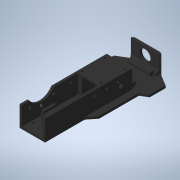
# Autodesk Inventor part: Griff_rechts
Saved by Autodesk Inventor 2021 (Build 250183000, 183)
## iProperties
Created: 2021-03-07
Part Number: Griff_rechts
Material: Generic
Document SubType Name: Modeling
Designer: Lukas
Density: 1 g/cm^3
Appearance: Default
Author: Lukas
Autodesk Inventor part; units mm, degrees
ref_plane "YZ Plane" through (0, 0, 0) normal (1, 0, 0) x (0, 1, 0)
ref_plane "XZ Plane" through (0, 0, 0) normal (0, 1, 0) x (-1, 0, 0)
ref_plane "XY Plane" through (0, 0, 0) normal (0, 0, 1) x (1, 0, 0)
sketch "Sketch27" plane through (0, 0, 0) normal (0, 1, 0) x (-1, 0, 0)
  line L0 (16, 72.5) -> (-16, 72.5)
  line L1 (-16, 72.5) -> (-16, -32.5)
  line L2 (16, -32.5) -> (16, 72.5)
  line L3 (16, -32.5) -> (32.5, -42.5)
  line L4 (32.5, -42.5) -> (32.5, -62.5)
  line L5 (32.5, -62.5) -> (16, -72.5)
  line L6 (16, -72.5) -> (-16, -72.5)
  line L7 (-16, -72.5) -> (-32.5, -62.5)
  line L8 (-32.5, -62.5) -> (-32.5, -42.5)
  line L9 (-32.5, -42.5) -> (-16, -32.5)
  circle A0 centre (0, -52.5) radius 1.6
  point P0 (0, 0)
  point P1 (0, -72.5)
  point P2 (0, 72.5)
  point P3 (-32.5, -52.5)
  dimension "d198" = 32
  dimension "d199" = 65
  dimension "d200" = 40
  dimension "d201" = 20
  dimension "d202" = 145
  dimension "d203" = 72.5
  dimension "d206" = 3.2
  constraints: 20 end point, 4 horizontal alignment, 4 vertical alignment, 3 midpoint, 3 perpendicular, 2 equal length, 1 centre point, 1 horizontal, 1 parallel, 1 vertical
  measures "d198" distance between parallel lines of L1 L2
  measures "d199" distance between parallel lines of L8 L4
  measures "d200" distance of L6.end L1.end
  measures "d201" distance of L7.end L8.end
  measures "d202" distance between parallel lines of L6 L0
  measures "d203" distance from line of point (0, 0) L0
  measures "d206" diameter of A0
extrude "Extrusion27" add sketch "Sketch27" along normal blind 3
sketch "Sketch28" plane through (0, 0, 0) normal (1, 0, 0) x (0, 1, 0)
  line L0 (3, -42.5) -> (3, -62.5) projected
  line L1 (3, -63) -> (8, -60)
  line L2 (8, -60) -> (8, -68)
  line L3 (0, -62.5) -> (0, -72.5) projected
  line L4 (8, -68) -> (3, -68)
  line L5 (3, -37) -> (8, -37)
  line L6 (8, -37) -> (8, -45)
  line L7 (8, -45) -> (3, -42)
  line L8 (3, -42) -> (3, -37)
  line L9 (3, -63) -> (3, -68)
  line L10 (3, -50.9) -> (3, -54.1) projected
  point P0 (0, 0)
  point P1 (3, -52.5)
  dimension "d207" = 15
  dimension "d208" = 21
  dimension "d209" = 8
  dimension "d210" = 7.5
  dimension "d211" = 5
  constraints: 16 end point, 8 point on line, 4 perpendicular, 2 equal length, 1 midpoint, 1 parallel
  measures "d207" distance of L6.end L1.end
  measures "d208" distance of L1.start L7.end
  measures "d209" distance of L1.end L2.end
  measures "d210" vertical distance of L1.end point (3, -52.5)
  measures "d211" horizontal distance of L1.start L1.end
extrude "Extrusion28" add sketch "Sketch28" along normal mid plane 28.25
sketch "Sketch29" plane through (0, 3, 0) normal (0, 1, 0) x (1, 0, 0)
  line L0 (-13, -69.5) -> (13, -69.5)
  line L1 (13, -69.5) -> (13, 37)
  line L2 (14.125, 37) -> (-14.125, 37) projected
  line L3 (-13, -69.5) -> (-13, 37)
  line L4 (14.125, 37) -> (16, 37)
  line L5 (16, 37) -> (16, 32.5)
  line L6 (16, 32.5) -> (32.5, 42.5) projected
  line L7 (-14.125, 37) -> (-16, 37)
  line L8 (-16, 37) -> (-16, 32.5)
  line L9 (-32.5, 42.5) -> (-16, 32.5) projected
  line L10 (-32.5, 42.5) -> (-16, 32.5) projected
  line L11 (16, -72.5) -> (16, 32.5) projected
  line L12 (-16, 32.5) -> (-16, -72.5) projected
  line L13 (-16, -72.5) -> (16, -72.5) projected
  line L14 (-13, -69.5) -> (-13, -72.5)
  line L15 (13, -69.5) -> (13, -72.5)
  line L16 (-16, -72.5) -> (16, -72.5) projected
  point P0 (0, 0)
  dimension "d215" = 3
  dimension "d217" = 3
  dimension "d218" = 3
  constraints: 18 end point, 6 point on line, 3 horizontal, 2 collinear, 2 parallel, 2 perpendicular, 1 vertical
  measures "d215" distance between parallel lines of L11 L1
  measures "d217" distance between parallel lines of L12 L3
  measures "d218" distance between parallel lines of L13 L0
extrude "Extrusion29" add sketch "Sketch29" along normal blind 23 contours L14 L13 L12 L8 L7 L2 L3 | L1 L2 L4 L5 L11 L13 L15
sketch "Sketch33" plane through (0, 3, 0) normal (0, 1, 0) x (1, 0, 0)
  line L0 (8.1, 43.2) -> (-8.1, 43.2)
  line L1 (-8.1, 43.2) -> (-8.1, -2)
  line L2 (-8.1, -2) -> (8.1, -2)
  line L3 (8.1, -2) -> (8.1, 43.2)
  circle A0 centre (6, -8) radius 1.6
  circle A1 centre (-6, -8) radius 1.6
  point P0 (0, 0)
  point P1 (0, 43.2)
  point P2 (0, 43.2)
  point P3 (0, 43.2)
  dimension "d234" = 45.2
  dimension "d235" = 16.2
  dimension "d238" = 2
  dimension "d285" = 6
  dimension "d286" = 3.2
  dimension "d287" = 6
  dimension "d288" = 12
  constraints: 8 end point, 3 midpoint, 2 centre point, 2 parallel, 1 equal radius, 1 horizontal, 1 horizontal alignment, 1 perpendicular, 1 vertical alignment
  measures "d234" distance of L2.end L0.start
  measures "d235" distance of L1.end L2.end
  measures "d238" distance from line of L2 point (0, 0)
  measures "d285" distance from line of L2 A0.centre
  measures "d286" diameter of A0
  measures "d287" horizontal distance of A0.centre point (0, 0)
  measures "d288" distance of A1.centre A0.centre
extrude "Extrusion33" cut sketch "Sketch33" against normal through all both and the other way through all
chamfer "Chamfer5" distance 1.85 angle 45 4 edges at (8.1, 1.5, -43.2) (8.1, 6.5, -43.2) (-8.1, 6.5, -43.2) (-8.1, 1.5, -43.2)
sketch "Sketch34" plane through (8.1, 3, 2) normal (0, 0, -1) x (-1, 0, 0)
  line L0 (0, -3) -> (0, 0) projected
  line L1 (0, 0) -> (0, 21)
  line L2 (0, 0) -> (16.2, 0) projected
  line L3 (16.2, 0) -> (16.2, 21)
  line L4 (-4.9, 23) -> (21.1, 23)
  line L5 (0, 21) -> (16.2, 21)
  line L6 (21.1, 0) -> (21.1, 23) projected
  line L7 (-4.9, 0) -> (-4.9, 23) projected
  line L8 (21.1, 0) -> (-4.9, 0) projected
  point P0 (8.1, -3)
  dimension "d255" = 21
  constraints: 8 end point, 2 vertical, 1 horizontal
  measures "d255" distance of L0.end L1.end
extrude "Extrusion34" add sketch "Sketch34" along normal up to surface (39 mm away) contours L8 L7 L4 L6 L3 L5 L1
sketch "Sketch35" plane through (8.1, 0, -41.35) normal (-1, 0, 0) x (0, 0, 1)
  circle A0 centre (18.35, 13.5) radius 2.55
  line L0 (43.35, 0) -> (0, 0) projected
  line L1 (43.35, 0) -> (43.35, 3) projected
  circle A1 centre (18.35, 13.5) radius 2.75
  point P0 (41.35, 0)
  dimension "d247" = 13.5
  dimension "d248" = 5.1
  dimension "d249" = 25
  dimension "d252" = 5.5
  constraints: 2 centre point, 1 coincident
  measures "d247" distance from line of L0 A0.centre
  measures "d248" diameter of A0
  measures "d249" distance from line of A0.centre L1
  measures "d252" diameter of A1
extrude "Extrusion35" cut sketch "Sketch35" against normal through all contours A0
extrude "Extrusion36" cut sketch "Sketch35" against normal blind 1
mirror "Mirror1" about plane through (0, 0, 0) normal (1, 0, 0) of "Extrusion35", "Extrusion36"
sketch "Sketch41" plane through (0, 0, 0) normal (0, -1, 0) x (1, 0, 0)
  circle A0 centre (6, 31) radius 1.6
  circle A1 centre (-6, 31) radius 1.6
  circle A2 centre (6, 8) radius 1.6 projected
  point P0 (0, 0)
  dimension "d296" = 6
  dimension "d297" = 12
  dimension "d298" = 3.2
  dimension "d412" = 23
  constraints: 2 centre point, 1 equal radius, 1 horizontal alignment
  measures "d296" horizontal distance of point (0, 0) A0.centre
  measures "d297" distance of A1.centre A0.centre
  measures "d298" diameter of A0
  measures "d412" distance of A2.centre A0.centre
extrude "Extrusion42" cut sketch "Sketch41" against normal through all contours A0 | A1
sketch "Sketch43" plane through (0, 26, 0) normal (0, 1, 0) x (1, 0, 0)
  circle A0 centre (-12, 31.5) radius 1.4
  circle A1 centre (12, 31.5) radius 1.4
  circle A2 centre (-12, 2.5) radius 1.4
  circle A3 centre (12, 2.5) radius 1.4
  point P0 (0, 0)
  dimension "d314" = 2.8
  dimension "d315" = 12
  dimension "d316" = 24
  dimension "d317" = 2.5
  dimension "d318" = 31.5
  constraints: 4 centre point, 3 equal radius, 2 horizontal alignment, 2 vertical alignment
  measures "d314" diameter of A0
  measures "d315" horizontal distance of point (0, 0) A0.centre
  measures "d316" distance of A0.centre A1.centre
  measures "d317" vertical distance of point (0, 0) A3.centre
  measures "d318" vertical distance of A1.centre point (0, 0)
extrude "Extrusion44" cut sketch "Sketch43" against normal through all
sketch "Sketch44" plane through (0, 3, 0) normal (0, 1, 0) x (1, 0, 0)
  line L0 (14.125, 68) -> (14.125, 63) projected
  line L1 (14.125, 68) -> (17.125, 68)
  line L2 (17.125, 68) -> (18.8174, 70.7925)
  line L3 (32.5, 62.5) -> (16, 72.5) projected
  line L4 (-14.125, 63) -> (-14.125, 68) projected
  line L5 (-14.125, 68) -> (-17.125, 68)
  line L6 (-17.125, 68) -> (-18.8174, 70.7925)
  line L7 (-16, 72.5) -> (-32.5, 62.5) projected
  line L8 (16, 72.5) -> (-16, 72.5) projected
  line L9 (-14.125, 68) -> (14.125, 68) projected
  line L10 (17.7311, 69) -> (-17.7311, 69)
  point P0 (0, 0)
  dimension "d321" = 3
  dimension "d322" = 3
  dimension "d355" = 3.5
  constraints: 10 end point, 5 point on line, 2 horizontal, 2 perpendicular
  measures "d321" distance of L0.start L1.end
  measures "d322" distance of L4.end L5.end
  measures "d355" distance between parallel lines of L8 L10
extrude "Extrusion45" add sketch "Sketch44" along normal up to surface (23 mm away) contours L10 L6 L7 L8 L3 L2
chamfer "Chamfer8" distance 6 angle 45 1 edges at (0, 3, -69)
sketch "Sketch45" plane through (16, 0, -72.5) normal (0, 0, -1) x (-1, 0, 0)
  circle A0 centre (16, 16) radius 7
  line L0 (32, 26) -> (0, 26) projected
  line L1 (1.875, 3) -> (30.125, 3) projected
  point P0 (16, 0)
  point P1 (16, 26)
  dimension "d325" = 13
  dimension "d326" = 14
  constraints: 1 centre point, 1 midpoint, 1 vertical alignment
  measures "d325" distance from line of A0.centre L1
  measures "d326" diameter of A0
extrude "Extrusion46" cut sketch "Sketch45" against normal blind 10
sketch "Sketch46" plane through (0, 3, 0) normal (0, 1, 0) x (1, 0, 0)
  circle A0 centre (10, -47.5) radius 1.6
  circle A1 centre (10, -61.5) radius 1.6
  circle A2 centre (-10, -47.5) radius 1.6
  circle A3 centre (-10, -61.5) radius 1.6
  line L0 (-13, -72.5) -> (13, -72.5) projected
  point P0 (0, 0)
  dimension "d329" = 3.2
  dimension "d331" = 10
  dimension "d332" = 20
  dimension "d333" = 14
  dimension "d424" = 11
  constraints: 4 centre point, 3 equal radius, 2 horizontal alignment, 2 vertical alignment
  measures "d329" diameter of A2
  measures "d331" horizontal distance of point (0, 0) A3.centre
  measures "d332" distance of A1.centre A3.centre
  measures "d333" distance of A2.centre A3.centre
  measures "d424" distance from line of L0 A1.centre
extrude "Extrusion47" cut sketch "Sketch46" against normal through all
sketch "Sketch47" plane through (13, 26, 69.5) normal (0, 0, -1) x (-1, 0, 0)
  circle A0 centre (5, -9) radius 1.6
  circle A1 centre (21, -9) radius 1.6
  line L0 (26, -23) -> (0, -23) projected
  point P0 (13, -26)
  point P1 (8, -23)
  dimension "d336" = 8
  dimension "d337" = 8
  dimension "d338" = 14
  dimension "d339" = 3.2
  constraints: 2 centre point, 1 equal radius, 1 horizontal alignment
  measures "d336" horizontal distance of point (13, -26) A1.centre
  measures "d337" horizontal distance of A0.centre point (13, -26)
  measures "d338" distance from line of L0 A0.centre
  measures "d339" diameter of A0
extrude "Extrusion48" [suppressed]
sketch "Sketch48" plane through (0, 0, 0) normal (0, -1, 0) x (1, 0, 0)
  line L0 (16, -32.5) -> (32.5, -42.5) projected
  line L1 (16, 72.5) -> (16, -32.5) projected
  line L2 (-16, -32.5) -> (-16, 72.5) projected
  line L3 (-32.5, -42.5) -> (-16, -32.5) projected
  line L4 (24, -37.3485) -> (24, 12.6515)
  line L5 (24, 12.6515) -> (16, 22.6515)
  line L6 (-16, 22.6515) -> (-24, 12.6515)
  line L7 (-24, 12.6515) -> (-24, -37.3485)
  line L8 (-32.5, -42.5) -> (-16, -32.5) projected
  point P0 (0, 0)
  point P1 (-24, -37.3485)
  dimension "d342" = 8
  dimension "d343" = 50
  dimension "d344" = 10
  constraints: 8 end point, 4 point on line, 2 equal length, 2 vertical, 1 horizontal alignment
  measures "d342" distance between parallel lines of L1 L4
  measures "d343" distance of L4.start L4.end
  measures "d344" vertical distance of L4.end L5.end
extrude "Extrusion49" add sketch "Sketch48" against normal up to surface (3 mm away)
sketch "Sketch49" plane through (16, 0, 72.5) normal (1, 0, 0) x (0, 0, -1)
  circle A0 centre (77.5, 20) radius 1.4
  line L0 (0, 26) -> (109.5, 26) projected
  line L1 (109.5, 3) -> (109.5, 26) projected
  circle A1 centre (91.5, 20) radius 1.4
  circle A2 centre (61.5, 20) radius 1.4
  point P0 (72.5, 0)
  dimension "d347" = 2.8
  dimension "d348" = 6
  dimension "d352" = 14
  dimension "d353" = 18
  dimension "d354" = 16
  constraints: 3 centre point, 2 equal radius, 2 horizontal alignment
  measures "d347" diameter of A0
  measures "d348" distance from line of L0 A0.centre
  measures "d352" distance of A1.centre A0.centre
  measures "d353" distance from line of L1 A1.centre
  measures "d354" distance of A0.centre A2.centre
extrude "Extrusion50" cut sketch "Sketch49" against normal blind 7
mirror "Mirror3" about plane through (0, 0, 0) normal (1, 0, 0) of "Extrusion50"
sketch "Sketch52" plane through (0, 0, 0) normal (0, -1, 0) x (1, 0, 0)
  circle A0 centre (0, -67.5) radius 1.4
  line L0 (16, -72.5) -> (-16, -72.5) projected
  point P0 (0, 0)
  point P1 (0, -72.5)
  dimension "d370" = 2.8
  dimension "d371" = 5
  constraints: 1 centre point, 1 midpoint, 1 vertical alignment
  measures "d370" diameter of A0
  measures "d371" distance from line of L0 A0.centre
extrude "Extrusion53" cut sketch "Sketch52" against normal blind 7
sketch "Sketch59" plane through (0, 3, 0) normal (0, 1, 0) x (1, 0, 0)
  line L0 (-6, -55.5) -> (6, -55.5)
  line L1 (6, -55.5) -> (6, -39.5)
  line L2 (6, -39.5) -> (-6, -39.5)
  line L3 (-6, -39.5) -> (-6, -55.5)
  line L4 (-13, -72.5) -> (13, -72.5) projected
  point P0 (0, 0)
  point P1 (0, -39.5)
  dimension "d413" = 12
  dimension "d414" = 16
  dimension "d415" = 17
  constraints: 8 end point, 2 parallel, 1 horizontal, 1 midpoint, 1 perpendicular, 1 vertical alignment
  measures "d413" distance of L1.end L2.end
  measures "d414" distance of L0.end L1.end
  measures "d415" distance between parallel lines of L4 L0
extrude "Extrusion60" add sketch "Sketch59" along normal blind 12.75
sketch "Sketch60" plane through (0, 15.75, 0) normal (0, 1, 0) x (1, 0, 0)
  line L0 (6, -39.5) -> (-6, -39.5) projected
  line L1 (-6, -55.5) -> (6, -55.5) projected
  line L2 (-3.05, -39.5) -> (3.05, -39.5)
  line L3 (3.05, -39.5) -> (3.05, -55.5)
  line L4 (3.05, -55.5) -> (-3.05, -55.5)
  line L5 (-3.05, -55.5) -> (-3.05, -39.5)
  point P0 (0, 0)
  point P1 (0, -39.5)
  point P2 (0, -39.5)
  dimension "d418" = 6.1
  constraints: 8 end point, 2 midpoint, 2 parallel, 2 point on line, 1 coincident, 1 horizontal, 1 perpendicular
  measures "d418" distance between parallel lines of L3 L5
extrude "Extrusion61" cut sketch "Sketch60" against normal blind 2.85
sketch "Sketch54" plane through (-16, 3, 69.5) normal (1, 0, 0) x (0, 0, -1)
  circle A0 centre (22, 32) radius 17.5
  line L0 (-3, -3) -> (-3, 23) projected
  line L1 (106.5, 23) -> (-3, 23) projected
  circle A1 centre (37, 15.9065) radius 1.6
  line L2 (21.6336, 10.9305) -> (22.3664, 9.0695) construction
  line L3 (20.1449, 10.3442) -> (20.8776, 8.4833)
  line L4 (23.8551, 9.6558) -> (23.1224, 11.5167)
  arc A2 (23.1224, 11.5167) -> (20.1449, 10.3442) centre (21.6336, 10.9305) ccw
  arc A3 (20.8776, 8.4833) -> (23.8551, 9.6558) centre (22.3664, 9.0695) ccw
  line L5 (7, 16.9065) -> (7, 14.9065) construction
  line L6 (5.4, 16.9065) -> (5.4, 14.9065)
  line L7 (8.6, 14.9065) -> (8.6, 16.9065)
  arc A4 (8.6, 16.9065) -> (5.4, 16.9065) centre (7, 16.9065) ccw
  arc A5 (5.4, 14.9065) -> (8.6, 14.9065) centre (7, 14.9065) ccw
  line L8 (22, 10) -> (23.4887, 10.5862)
  line L9 (7, 15.9065) -> (8.6, 15.9065)
  point P0 (69.5, -3)
  dimension "d374" = 25
  dimension "d375" = 35
  dimension "d376" = 9
  dimension "d427" = 22
  dimension "d430" = 15
  dimension "d431" = 3.2
  dimension "d432" = 22
  dimension "d433" = 22
  dimension "d434" = 2
  constraints: 20 end point, 8 point on circle, 8 tangent, 6 centre point, 4 midpoint, 2 equal radius, 2 parallel, 2 point on line, 1 equal length, 1 horizontal alignment, 1 vertical alignment
  measures "d374" distance from line of L0 A0.centre
  measures "d375" diameter of A0
  measures "d376" distance from line of L1 A0.centre
  measures "d427" distance of A0.centre A1.centre
  measures "d430" horizontal distance of A0.centre A1.centre
  measures "d431" diameter of A1
  measures "d432" distance of L9.start A0.centre
  measures "d433" distance of L8.start A0.centre
  measures "d434" distance of L3.start L3.end
extrude "Extrusion54" cut sketch "Sketch54" along normal blind 4
body "Solid3"
